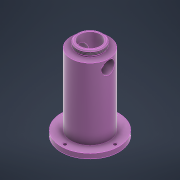
# Autodesk Inventor part: 013
Saved by Autodesk Inventor 2022 (Build 260153000, 153)
## iProperties
Created: 2021-11-02
Part Number: 013
Material: Stainless Steel, Austenitic
Document SubType Name: Modeling
Designer: vinicius.miguel
Density: 8 g/cm^3
Appearance: Smooth - Purple
Mass: 322.499 g
Surface Area: 186.589 cm^2
Volume: 40.3124 cm^3
Author: vinicius.miguel
Autodesk Inventor part; units mm, degrees
ref_plane "XZ Plane" through (0, 0, 0) normal (0, 1, 0) x (-1, 0, 0)
ref_plane "XY Plane" through (0, 0, 0) normal (0, 0, 1) x (1, 0, 0)
sketch "Sketch1" plane through (0, 0, 0) normal (0, 0, 1) x (1, 0, 0)
  line L0 (0, 0) -> (0, 82.5)
  line L1 (11, 82.5) -> (12, 81.5)
  line L2 (12, 81.5) -> (12, 78.5)
  line L3 (12, 78.5) -> (11, 77.5)
  line L4 (11, 77.5) -> (11, 76.5)
  line L5 (11, 76.5) -> (17.5, 76.5)
  line L6 (17.5, 76.5) -> (17.5, 11)
  line L7 (17.5, 11) -> (26.5, 11)
  line L8 (26.5, 11) -> (26.5, 6.5)
  line L9 (15, 0) -> (13, 0)
  line L10 (13, 0) -> (13, 56)
  line L11 (13, 56) -> (4, 56)
  line L12 (9.5, 62.5) -> (9.5, 82.5)
  line L13 (9.5, 82.5) -> (11, 82.5)
  line L14 (9.5, 62.5) -> (9, 62.5)
  line L15 (9, 62.5) -> (9, 61)
  line L16 (10, 59) -> (6.4, 59)
  line L17 (-4, 47) -> (4, 47)
  line L18 (4, 47) -> (4, 45)
  line L19 (4, 45) -> (-4, 45)
  line L20 (-4, 45) -> (-4, 47)
  line L21 (-4, 47) -> (4, 45) construction
  line L22 (4, 47) -> (-4, 45) construction
  line L23 (9, 61) -> (10, 61)
  line L24 (10, 61) -> (10, 59)
  line L25 (4, 56) -> (4, 56.6)
  line L26 (4, 56.6) -> (6.4, 59)
  circle A0 centre (5, 59) radius 1
  line L27 (26.5, 6.5) -> (13, 6.5)
  point P0 (0, 46)
  dimension "d0" = 26
  dimension "d1" = 35
  dimension "d8" = 56
  dimension "d11" = 24
  dimension "d14" = 135
  dimension "d15" = 22
  dimension "d16" = 22
  dimension "d18" = 3
  dimension "d22" = 19
  dimension "d26" = 135
  dimension "d28" = 6
  dimension "d30" = 18
  dimension "d38" = 8
  dimension "d39" = 2
  dimension "d50" = 14
  dimension "d59" = 20
  dimension "d60" = 2
  dimension "d61" = 3.5
  dimension "d62" = 0.6
  dimension "d63" = 3
  dimension "d64" = 2
  dimension "d65" = 10
  dimension "d66" = 8
  dimension "d67" = 135
  dimension "d68" = 53
  dimension "d69" = 11
  dimension "d70" = 4.5
  constraints: 56 end point, 10 perpendicular, 3 horizontal, 3 parallel, 3 vertical, 2 horizontal alignment, 2 midpoint, 2 point on line, 1 centre point
  measures "d0" diameter of L10 L0
  measures "d1" diameter of L6 L0
  measures "d8" distance from line of L11 L0.start
  measures "d11" diameter of L2 L0
  measures "d14" angle of L3 L2
  measures "d15" diameter of L1.start L0
  measures "d16" diameter of L4 L0
  measures "d18" distance of L1.end L2.end
  measures "d22" diameter of L12 L0
  measures "d26" angle of L13 L1
  measures "d28" distance from line of L5 L0.end
  measures "d30" diameter of L15 L0
  measures "d38" distance of L18.end L19.end
  measures "d39" distance of L17.end L18.end
  measures "d50" distance between parallel lines of L5 L14
  measures "d59" diameter of L24 L0
  measures "d60" distance of L16.start L23.end
  measures "d61" distance between parallel lines of L14 L16
  measures "d62" distance of L11.end L25.end
  measures "d63" distance between parallel lines of L11 L16
  measures "d64" diameter of A0
  measures "d65" diameter of A0.centre L0
  measures "d66" diameter of L25 L0
  measures "d67" angle of L26 L16
  measures "d68" diameter of L8 L0
  measures "d69" distance from line of L7 L0.start
  measures "d70" distance of L7.end L8.end
revolve "Revolution1" add sketch "Sketch1" angle 360 about axis through (0, 0, 0) along (0, 1, 0) picked at (5.7132, 58.309) contours L1 L2 L3 L4 L5 L6 L7 L8 L27 L10 L11 L25 L26 A0 L16 L24 L23 L15 L14 L12 L13 | A0 L26
ref_plane "Work Plane1" through (18.5, 0, 0) normal (1, 0, 0) x (0, 1, 0)
sketch "Sketch2" plane through (18.5, 0, 0) normal (1, 0, 0) x (0, 1, 0)
  line L0 (76.5, 17.5) -> (76.5, -17.5) projected
  point P0 (0, 0)
  point P1 (69.5, 0)
  point P2 (76.5, 0)
  dimension "d41" = 7
  constraints: 1 horizontal alignment, 1 midpoint
  measures "d41" distance from line of point (69.5, 0) L0
hole "Hole1" at (18.5, 69.5, 0) direction (-1, 0, 0) diameter 12 end through all
thread "Thread1" size "M24x1" class "6g" standard "ANSI Metric M Profile" full length
thread "Thread2" size "M18x0.5" class "6H" standard "ANSI Metric M Profile" full length
sketch "Sketch3" plane through (0, 6.5, 0) normal (0, -1, 0) x (1, 0, 0)
  point P0 (0, 0)
  point P1 (23, 0)
  dimension "d71" = 23
  constraints: 1 horizontal alignment
  measures "d71" distance of point (23, 0) point (0, 0)
hole "Hole2" at (23, 6.5, 0) direction (0, 1, 0) diameter 3.1 end through all clearance for "Countersunk Flat Head Screw DIN EN ISO 2009" size "M2.5" standard "DIN"
pattern_circular "Circular Pattern1" count 4 over 360 about axis through (0, 43.75, 0) along (0, -1, 0) of "Hole2"
sketch "Sketch4" plane through (0, 6.5, 0) normal (0, -1, 0) x (1, 0, 0)
  circle A0 centre (0, 0) radius 13 projected
  circle A1 centre (0, 0) radius 18.5983
  constraints: 1 centre point
extrude "Extrusion1" add sketch "Sketch4" along normal blind 3.5
sketch "Sketch5" plane through (0, 3, 0) normal (0, -1, 0) x (1, 0, 0)
  circle A0 centre (0, 0) radius 18.5983 projected
  circle A1 centre (0, 0) radius 13 projected
  circle A2 centre (0, 0) radius 13 projected
  line L0 (0, 13) -> (0, 18.5983)
  circle A3 centre (0, 0) radius 18.5983 projected
  line L1 (0, -18.5983) -> (0, -13)
  point P0 (0, 0)
  point P1 (0, 15.7991)
  point P2 (0, -15.7991)
  constraints: 4 end point, 4 vertical alignment, 2 midpoint, 2 point on line, 1 point on circle, 1 vertical, 3 other
hole "Hole3" at (0, 3, 15.7991) at (0, 3, -15.7991) direction (0, 1, 0) diameter 2.013 depth 5 tip angle 118 thread size "M2.5x0.45" class "6H" standard "ISO Metric profile"
equation "\"d14\" = d13"
equation "\"d13\" = 135deg"
body "Solid1"
